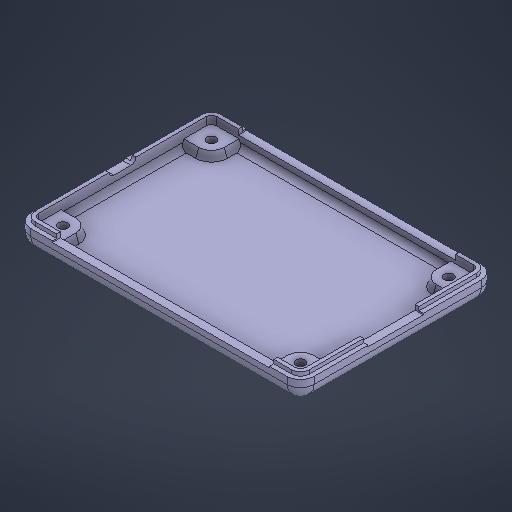
# Autodesk Inventor part: case1
Saved by Autodesk Inventor 2025.2 (Build 292293000, 293)
## iProperties
Created: 2025-10-04
Part Number: case1
Material: Generic
Document SubType Name: Modeling
Designer: micyg
Density: 1 g/cm^3
Appearance: Default
Author: micyg
## iProperties of the stored document case1_3DPrint.ipt
Created: 2025-10-05
Part Number: case1_3DPrint
Material: Generic
Document SubType Name: Modeling
Designer: micyg
Density: 1 g/cm^3
Appearance: Default
Author: micyg
Autodesk Inventor part; units mm, degrees
ref_plane "YZ Plane" through (0, 0, 0) normal (1, 0, 0) x (0, 1, 0)
ref_plane "XZ Plane" through (0, 0, 0) normal (0, 1, 0) x (-1, 0, 0)
ref_plane "XY Plane" through (0, 0, 0) normal (0, 0, 1) x (1, 0, 0)
sketch "Sketch1" plane through (0, 0, 0) normal (0, 1, 0) x (-1, 0, 0)
  line L0 (0, 0) -> (105, 0)
  line L1 (105, 0) -> (105, -72)
  line L2 (105, -72) -> (0, -72)
  line L3 (0, -72) -> (0, 0)
  line L4 (0, -72) -> (105, 0) construction
  line L5 (3.5, -3.5) -> (101.5, -3.5) construction
  line L6 (101.5, -3.5) -> (101.5, -68.5) construction
  line L7 (101.5, -68.5) -> (3.5, -68.5) construction
  line L8 (3.5, -68.5) -> (3.5, -3.5) construction
  line L9 (3.5, -3.5) -> (101.5, -68.5) construction
  line L10 (101.5, -3.5) -> (3.5, -68.5) construction
  point P0 (52.5, -36)
  dimension "d17" = 98
  dimension "d18" = 65
  dimension "d21" = 72
  dimension "d22" = 105
  constraints: 22 end point, 4 parallel, 3 midpoint, 2 horizontal, 2 perpendicular
  measures "d17" distance of L6.end L7.end
  measures "d18" distance of L5.end L6.end
  measures "d21" distance between parallel lines of L2 L0
  measures "d22" distance between parallel lines of L3 L1
extrude "Extrusion1" add sketch "Sketch1" along normal blind 7.6
fillet "Fillet3" radius 5 4 edges at (-105, 3.8, -72) (-105, 3.8, 0) (0, 3.8, -72) (0, 3.8, 0)
fillet "Fillet6" radius 5 8 edges at (-1.4645, 0, -70.5355) (-52.5, 0, -72) (-103.5355, 0, -70.5355) (-105, 0, -36) (-103.5355, 0, -1.4645) (-52.5, 0, 0) (-1.4645, 0, -1.4645) (0, 0, -36)
shell "Shell2" thickness 3 removed faces 1 at (-36.6667, 7.6, -48)
sketch "Sketch2" plane through (-100, 3, -69) normal (0, 1, 0) x (1, 0, 0)
  line L0 (91.5, -5.5) -> (3.5, -5.5) construction
  line L1 (3.5, -5.5) -> (3.5, -60.5) construction
  line L2 (3.5, -60.5) -> (91.5, -60.5) construction
  line L3 (91.5, -60.5) -> (91.5, -5.5) construction
  arc A0 (91.5, -55.75) -> (86.75, -60.5) centre (91.5, -60.5) ccw
  line L4 (95, 0) -> (0, 0) construction
  arc A1 (-2, -64) -> (0, -66) centre (0, -64) ccw projected
  line L5 (-2, -64) -> (-2, -2) projected
  arc A2 (0, 0) -> (-2, -2) centre (0, -2) ccw projected
  line L6 (0, 0) -> (95, 0) projected
  arc A3 (97, -2) -> (95, 0) centre (95, -2) ccw projected
  line L7 (97, -2) -> (97, -64) projected
  arc A4 (95, -66) -> (97, -64) centre (95, -64) ccw projected
  line L8 (95, -66) -> (0, -66) projected
  arc A5 (95, -69) -> (100, -64) centre (95, -64) ccw projected
  line L9 (100, -64) -> (100, -2) projected
  arc A6 (100, -2) -> (95, 3) centre (95, -2) ccw projected
  line L10 (95, 3) -> (0, 3) projected
  arc A7 (0, 3) -> (-5, -2) centre (0, -2) ccw projected
  line L11 (-5, -2) -> (-5, -64) projected
  arc A8 (-5, -64) -> (0, -69) centre (0, -64) ccw projected
  line L12 (0, -69) -> (95, -69) projected
  line L13 (91.5, -55.75) -> (97, -55.75)
  line L14 (86.75, -60.5) -> (86.75, -66)
  circle A9 centre (91.5, -60.5) radius 1.75
  line L15 (-5, -2) -> (-5, -64) projected
  line L16 (-5, -33) -> (100, -33) construction
  line L17 (47.5, -69) -> (47.5, 3) construction
  line L18 (3.5, -60.5) -> (91.5, -5.5) construction
  point P0 (100, -69)
  point P1 (47.5, -33)
  dimension "d13" = 88
  dimension "d14" = 55
  dimension "d25" = 3.5
  dimension "d26" = 3
  constraints: 18 end point, 6 midpoint, 4 point on line, 2 centre point, 2 coincident, 2 parallel, 2 perpendicular, 2 point on circle, 1 horizontal, 1 tangent
  measures "d13" distance between parallel lines of L1 L3
  measures "d14" distance of L2.end L0.start
  measures "d25" diameter of A9
  measures "d26" radial gap between concentric circles of A0 A9
extrude "Extrusion2" add sketch "Sketch2" along normal blind 3 contours L13 L7 A4 L8 L14 A0
ref_plane "Work Plane1" through (-52.5, 7.6, -3) normal (-1, 0, 0) x (0, -1, 0)
ref_plane "Work Plane2" through (-3, 7.6, -36) normal (0, 0, 1) x (1, 0, 0)
sketch "Sketch3" plane through (-8.5, 3, -8.5) normal (0, 1, 0) x (1, 0, 0)
  circle A0 centre (0, 0) radius 1.75 projected
  point P0 (8.5, -8.5)
extrude "Extrusion3" cut sketch "Sketch3" against normal up to surface (3 mm away)
ref_plane "Work Plane3" through (-8.5, 0, -8.5) normal (0, 0, -1) x (-1, 0, 0)
sketch "Sketch4" plane through (-8.5, 0, -8.5) normal (0, 0, -1) x (-1, 0, 0)
  line L0 (1.75, 0) -> (-1.75, 0) projected
  line L1 (-1.75, 6) -> (1.75, 6) projected
  line L2 (-3.5, 0) -> (91.5, 0) projected
  line L3 (0, 0) -> (-3, 0)
  line L4 (-3, 0) -> (-3, 3)
  line L5 (-3, 3) -> (0, 3)
  line L6 (0, 3) -> (0, 0)
  line L7 (0, 3) -> (-3, 2)
  point P0 (-8.5, 0)
  point P1 (-3, 0)
  dimension "d30" = 3
  dimension "d31" = 3
  dimension "d32" = 1
  constraints: 10 end point, 2 parallel, 2 point on line, 1 horizontal, 1 midpoint, 1 perpendicular
  measures "d30" distance between parallel lines of L2 L5
  measures "d31" distance between parallel lines of L6 L4
  measures "d32" distance from line of L5 L7.end
revolve "Revolution1" cut sketch "Sketch4" angle 360 about axis through (-8.5, 3, -8.5) along (0, -1, 0) contours L0 L2 L4 L7 L6
draft "FaceDraft1" angle 20 pull direction (0, 1, 0) faces at (-10.2354, 5, -12.9217) (-13.25, 5, -5.5) (-5.5, 5, -13.25) fixed edges at (-11.8588, 6, -11.8588) (-13.25, 6, -5.75) (-5.75, 6, -13.25)
mirror "Mirror3" about plane through (-3, 7.6, -36) normal (0, 0, 1) of "Extrusion2", "Extrusion3", "Revolution1", "FaceDraft1"
mirror "Mirror4" about plane through (-52.5, 7.6, -3) normal (-1, 0, 0) of "Extrusion2", "Extrusion3", "Mirror3", "FaceDraft1", "Revolution1"
sketch "Sketch5" plane through (0, 7.6, 0) normal (0, 1, 0) x (1, 0, 0)
  arc A0 (-100, 69) -> (-102, 67) centre (-100, 67) ccw projected
  line L0 (-100, 69) -> (-5, 69) projected
  arc A1 (-3, 67) -> (-5, 69) centre (-5, 67) ccw projected
  line L1 (-3, 67) -> (-3, 5) projected
  arc A2 (-5, 3) -> (-3, 5) centre (-5, 5) ccw projected
  line L2 (-5, 3) -> (-100, 3) projected
  arc A3 (-102, 5) -> (-100, 3) centre (-100, 5) ccw projected
  line L3 (-102, 5) -> (-102, 67) projected
  arc A4 (-5, 0) -> (0, 5) centre (-5, 5) ccw projected
  line L4 (0, 5) -> (0, 67) projected
  arc A5 (0, 67) -> (-5, 72) centre (-5, 67) ccw projected
  line L5 (-5, 72) -> (-100, 72) projected
  arc A6 (-100, 72) -> (-105, 67) centre (-100, 67) ccw projected
  line L6 (-105, 67) -> (-105, 5) projected
  arc A7 (-105, 5) -> (-100, 0) centre (-100, 5) ccw projected
  line L7 (-100, 0) -> (-5, 0) projected
  arc A8 (-100, 70.4) -> (-103.4, 67) centre (-100, 67) ccw
  line L8 (-100, 70.4) -> (-5, 70.4)
  arc A9 (-1.6, 67) -> (-5, 70.4) centre (-5, 67) ccw
  line L9 (-1.6, 67) -> (-1.6, 5)
  arc A10 (-5, 1.6) -> (-1.6, 5) centre (-5, 5) ccw
  line L10 (-5, 1.6) -> (-100, 1.6)
  arc A11 (-103.4, 5) -> (-100, 1.6) centre (-100, 5) ccw
  line L11 (-103.4, 5) -> (-103.4, 67)
  point P0 (0, 0)
  dimension "d35" = 1.4
  constraints: 8 end point, 8 point on circle, 4 centre point, 7 other
  measures "d35" distance between parallel lines of L3 L11
extrude "Extrusion4" add sketch "Sketch5" along normal blind 1.4 contours L8 A9 L9 A10 L10 A11 L11 A8
sketch "Sketch6" plane through (-3, 6, -13.25) normal (-1, 0, 0) x (0, 0, 1)
  line L0 (-12.25, 1.595) -> (-12.25, 21.095) projected
  line L1 (-31.75, 1.595) -> (-12.25, 1.595) projected
  line L2 (-31.75, 1.595) -> (-31.75, 21.095) projected
  line L3 (-12.25, 21.095) -> (-31.75, 21.095) projected
  circle A0 centre (-22.75, 11.595) radius 7 projected
  line L4 (-53.75, 0) -> (-45.5, 0) projected
  line L5 (-45.5, 0) -> (-45.136, -1) projected
  line L6 (-45.136, -1) -> (-0.364, -1) projected
  line L7 (-0.364, -1) -> (0, 0) projected
  line L8 (0, 0) -> (8.25, 0) projected
  line L9 (8.25, 0) -> (8.25, 3) projected
  line L10 (-53.75, 3) -> (8.25, 3) projected
  line L11 (-53.75, 3) -> (-53.75, 0) projected
  line L12 (-11.75, 1.095) -> (-11.75, 21.595)
  line L13 (-11.75, 21.595) -> (-32.25, 21.595)
  line L14 (-32.25, 21.595) -> (-32.25, 1.095)
  line L15 (-32.25, 1.095) -> (-11.75, 1.095)
  point P0 (13.25, -6)
  dimension "d38" = 0.5
  constraints: 8 end point, 3 other
  measures "d38" distance between parallel lines of L1 L15
extrude "Extrusion5" cut sketch "Sketch6" against normal up to surface (3 mm away) contours L1 L2 L10 L0 | L0 L10 L12 L15 L14 L2 L1 | L10 L2 L3 L0 | L0 L3 L2 L10 L14 L13 L12 | A0
sketch "Sketch7" plane through (-13.25, 6, -69) normal (0, 0, 1) x (1, 0, 0)
  line L0 (-58.75, 1.595) -> (-58.75, 21.095) projected
  line L1 (-78.25, 1.595) -> (-58.75, 1.595) projected
  line L2 (-78.25, 1.595) -> (-78.25, 21.095) projected
  line L3 (-58.75, 21.095) -> (-78.25, 21.095) projected
  circle A0 centre (-69.25, 11.595) radius 7 projected
  line L4 (-38.75, 1.595) -> (-38.75, 21.095) projected
  line L5 (-58.25, 1.595) -> (-38.75, 1.595) projected
  line L6 (-58.25, 1.595) -> (-58.25, 21.095) projected
  line L7 (-38.75, 21.095) -> (-58.25, 21.095) projected
  circle A1 centre (-49.25, 11.595) radius 7 projected
  line L8 (-18.75, 1.595) -> (-18.75, 21.095) projected
  line L9 (-38.25, 1.595) -> (-18.75, 1.595) projected
  line L10 (-38.25, 1.595) -> (-38.25, 21.095) projected
  line L11 (-18.75, 21.095) -> (-38.25, 21.095) projected
  circle A2 centre (-29.25, 11.595) radius 7 projected
  line L12 (1.25, 1.595) -> (1.25, 21.095) projected
  line L13 (-18.25, 1.595) -> (1.25, 1.595) projected
  line L14 (-18.25, 1.595) -> (-18.25, 21.095) projected
  line L15 (1.25, 21.095) -> (-18.25, 21.095) projected
  circle A3 centre (-9.25, 11.595) radius 7 projected
  line L16 (-58.75, 1.595) -> (-58.75, 21.095) projected
  line L17 (-78.25, 1.595) -> (-58.75, 1.595) projected
  line L18 (-78.25, 1.595) -> (-78.25, 21.095) projected
  line L19 (-58.75, 21.095) -> (-78.25, 21.095) projected
  circle A4 centre (-69.25, 11.595) radius 7 projected
  line L20 (-86.75, 0) -> (-78.5, 0) projected
  line L21 (-78.5, 0) -> (-78.136, -1) projected
  line L22 (-78.136, -1) -> (-0.364, -1) projected
  line L23 (-0.364, -1) -> (0, 0) projected
  line L24 (0, 0) -> (8.25, 0) projected
  line L25 (8.25, 0) -> (8.25, 3) projected
  line L26 (-86.75, 3) -> (8.25, 3) projected
  line L27 (-86.75, 0) -> (-86.75, 3) projected
  line L28 (-78.75, 3) -> (1.75, 3)
  line L29 (1.75, 3) -> (1.75, 1.095)
  line L30 (1.75, 1.095) -> (-78.75, 1.095)
  line L31 (-78.75, 1.095) -> (-78.75, 3)
  point P0 (13.25, -6)
  point P1 (1.75, 3)
  dimension "d41" = 0.5
  dimension "d42" = 0.5
  dimension "d43" = 0.5
  constraints: 8 end point, 2 parallel, 1 horizontal, 1 perpendicular, 1 point on line
  measures "d41" distance between parallel lines of L13 L30
  measures "d42" distance between parallel lines of L12 L29
  measures "d43" distance between parallel lines of L31 L2
extrude "Extrusion6" cut sketch "Sketch7" against normal up to surface (3 mm away) contours L1 L2 L26 L0 | L0 L26 L6 L5 L4 L10 L9 L8 L14 L13 L12 L29 L30 L31 L2 L1 | L26 L4 L5 L6 | L26 L8 L9 L10 | L26 L12 L13 L14
mirror "Mirror5" about plane through (-3, 7.6, -36) normal (0, 0, 1) of "Extrusion6"
sketch "Sketch8" plane through (-102, 5, -13.614) normal (1, 0, 0) x (0, 0, -1)
  line L0 (22.386, 2.945) -> (22.386, 2.745) projected
  line L1 (19.196, 2.745) -> (22.386, 2.745) projected
  arc A0 (17.916, 4.025) -> (19.196, 2.745) centre (19.196, 4.025) ccw projected
  line L2 (17.916, 4.625) -> (17.916, 4.025) projected
  arc A1 (19.196, 5.905) -> (17.916, 4.625) centre (19.196, 4.625) ccw projected
  line L3 (22.386, 5.905) -> (19.196, 5.905) projected
  line L4 (22.386, 5.905) -> (22.386, 5.705) projected
  line L5 (22.386, 5.705) -> (19.196, 5.705) projected
  arc A2 (19.196, 5.705) -> (18.116, 4.625) centre (19.196, 4.625) ccw projected
  line L6 (18.116, 4.625) -> (18.116, 4.025) projected
  arc A3 (18.116, 4.025) -> (19.196, 2.945) centre (19.196, 4.025) ccw projected
  line L7 (19.196, 2.945) -> (22.386, 2.945) projected
  line L8 (22.386, 2.945) -> (22.386, 2.745) projected
  line L9 (25.576, 2.945) -> (22.386, 2.945) projected
  arc A4 (25.576, 2.945) -> (26.656, 4.025) centre (25.576, 4.025) ccw projected
  line L10 (26.656, 4.625) -> (26.656, 4.025) projected
  arc A5 (26.656, 4.625) -> (25.576, 5.705) centre (25.576, 4.625) ccw projected
  line L11 (22.386, 5.705) -> (25.576, 5.705) projected
  line L12 (22.386, 5.905) -> (22.386, 5.705) projected
  line L13 (22.386, 5.905) -> (25.576, 5.905) projected
  arc A6 (26.856, 4.625) -> (25.576, 5.905) centre (25.576, 4.625) ccw projected
  line L14 (26.856, 4.625) -> (26.856, 4.025) projected
  arc A7 (25.576, 2.745) -> (26.856, 4.025) centre (25.576, 4.025) ccw projected
  line L15 (25.576, 2.745) -> (22.386, 2.745) projected
  line L16 (22.386, 2.245) -> (19.196, 2.245)
  arc A8 (17.416, 4.025) -> (19.196, 2.245) centre (19.196, 4.025) ccw
  line L17 (17.416, 4.025) -> (17.416, 4.625)
  arc A9 (19.196, 6.405) -> (17.416, 4.625) centre (19.196, 4.625) ccw
  line L18 (19.196, 6.405) -> (22.386, 6.405)
  line L19 (22.386, 2.245) -> (25.576, 2.245)
  arc A10 (25.576, 2.245) -> (27.356, 4.025) centre (25.576, 4.025) ccw
  line L20 (27.356, 4.025) -> (27.356, 4.625)
  arc A11 (27.356, 4.625) -> (25.576, 6.405) centre (25.576, 4.625) ccw
  line L21 (25.576, 6.405) -> (22.386, 6.405)
  point P0 (-13.614, -5)
  dimension "d46" = 0.5
  constraints: 12 end point, 8 point on circle, 4 centre point, 8 other
  measures "d46" distance between parallel lines of L1 L16
extrude "Extrusion7" cut sketch "Sketch8" against normal up to surface (3 mm away) contours L9 A4 L10 A5 L11 L4 L13 A6 L14 A7 L15 L0 | L0 L1 A0 L2 A1 L3 L4 L5 A2 L6 A3 L7 | L7 A3 L6 A2 L5 L11 A5 L10 A4 L9 | L16 A8 L17 A9 L18 L21 A11 L20 A10 L19
equation "\"d29\" = d7"
equation "\"d42\" = d41"
equation "\"d43\" = d41"
equation "\"d7\" = 5"
body "Solid1"
